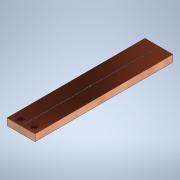
# Autodesk Inventor part: Leads+ChannelForSingleHeater
Saved by Autodesk Inventor 2021 (Build 250183000, 183)
## iProperties
Created: 2021-12-02
Part Number: Leads+ChannelForSingleHeater
Material: Generic
Document SubType Name: Sheet Metal
Designer: Unit-005
Density: 1 g/cm^3
Sheet Metal Rule: Default
Appearance: Default
Author: Unit-005
Autodesk Inventor part; units mm, degrees
ref_plane "YZ Plane" through (0, 0, 0) normal (1, 0, 0) x (0, 1, 0)
ref_plane "XZ Plane" through (0, 0, 0) normal (0, 1, 0) x (-1, 0, 0)
ref_plane "XY Plane" through (0, 0, 0) normal (0, 0, 1) x (1, 0, 0)
sketch "Sketch1" plane through (0, 0, 0) normal (0, 1, 0) x (-1, 0, 0)
  line L0 (-2.5781, 12.7) -> (2.5781, 12.7)
  line L1 (2.5781, 12.7) -> (2.5781, -12.7)
  line L2 (2.5781, -12.7) -> (-2.5781, -12.7)
  line L3 (-2.5781, -12.7) -> (-2.5781, 12.7)
  line L4 (-2.5781, 12.7) -> (2.5781, -12.7) construction
  line L5 (2.5781, 12.7) -> (-2.5781, -12.7) construction
  point P0 (0, 0)
  dimension "d0" = 5.1562
  dimension "d1" = 25.4
  constraints: 12 end point, 2 midpoint, 2 parallel, 1 horizontal, 1 perpendicular
  measures "d0" distance of L1.end L2.end
  measures "d1" distance of L0.end L1.end
extrude "Extrusion1" add sketch "Sketch1" along normal blind 1.1938
sketch "Sketch2" plane through (0, 1.1938, 0) normal (0, 1, 0) x (1, 0, 0)
  line L0 (2.5781, 12.7) -> (-2.5781, 12.7) projected
  line L1 (-2.5781, 12.7) -> (-2.5781, -12.7) projected
  line L2 (-2.5781, -12.7) -> (2.5781, -12.7) projected
  line L3 (2.5781, -12.7) -> (2.5781, 12.7) projected
  line L4 (-3.6093, 0) -> (3.6093, 0) projected
  line L5 (0, 17.78) -> (0, -17.78) projected
  circle A0 centre (1.27, -11.5062) radius 0.5969
  circle A1 centre (-1.27, -11.5062) radius 0.5969
  line L6 (2.5781, 12.7) -> (-2.5781, 12.7) projected
  line L7 (0.0508, -12.7) -> (-0.0508, -12.7)
  line L8 (-0.0508, -12.7) -> (-0.0508, 12.7)
  line L9 (-0.0508, 12.7) -> (0.0508, 12.7)
  line L10 (0.0508, 12.7) -> (0.0508, -12.7)
  line L11 (0.0508, -12.7) -> (-0.0508, 12.7) construction
  line L12 (-0.0508, -12.7) -> (0.0508, 12.7) construction
  point P0 (0, 0)
  dimension "d4" = 1.1938
  dimension "d5" = 1.1938
  dimension "d8" = 1.27
  dimension "d9" = 0.1016
  constraints: 12 end point, 2 centre point, 2 midpoint, 2 parallel, 1 horizontal, 1 perpendicular, 1 point on line, 1 symmetric about line, 1 other
  measures "d4" diameter of A0
  measures "d5" distance from line of L2 A0.centre
  measures "d8" distance from line of L5 A0.centre
  measures "d9" distance of L8.end L9.end
extrude "Extrusion2" add sketch "Sketch2" along normal blind 0.0381 contours L3 L4 L10 L0 | L3 L2 L10 L4 | L8 L4 L1 L0 | L8 L2 L1 L4
sketch "Sketch3" plane through (1.27, 1.1938, 11.5062) normal (0, 1, 0) x (1, 0, 0)
  point P0 (-1.27, 11.5062)
sketch "Sketch4" plane through (0, 0, 0) normal (0, 1, 0) x (-1, 0, 0)
  circle A0 centre (-1.27, 11.5062) radius 0.5969 projected
  circle A1 centre (1.27, 11.5062) radius 0.5969 projected
  line L0 (3.6093, 0) -> (-3.6093, 0) projected
  line L1 (0, -17.78) -> (0, 17.78) projected
  line L2 (0.0508, -12.7) -> (2.5781, -12.7) projected
  line L3 (2.5781, -12.7) -> (2.5781, 12.7) projected
  line L4 (2.5781, 12.7) -> (0.0508, 12.7) projected
  line L5 (0.0508, 12.7) -> (0.0508, -12.7) projected
  circle A2 centre (1.27, 11.5062) radius 0.5969 projected
  line L6 (-0.0508, 12.7) -> (-2.5781, 12.7) projected
  line L7 (-2.5781, 12.7) -> (-2.5781, -12.7) projected
  line L8 (-2.5781, -12.7) -> (-0.0508, -12.7) projected
  line L9 (-0.0508, -12.7) -> (-0.0508, 12.7) projected
  circle A3 centre (-1.27, 11.5062) radius 0.5969 projected
  point P0 (0, 0)
extrude "Extrusion3" cut sketch "Sketch4" along normal through all contours A0 | A1
equation "\"BendRadius\" = Thickness"
equation "\"BendReliefWidth\" = Thickness"
equation "\"BendReliefDepth\" = 0.5 * Thickness"
equation "\"CornerReliefSize\" = 4 * Thickness"
equation "\"MinimumRemnant\" = 2 * Thickness"
equation "\"TransitionRadius\" = BendRadius"
equation "\"JacobiRadiusSize\" = BendRadius"
equation "\"GapSize\" = Thickness"
equation "\"Thickness\" = 3.048"
body "Solid1"
